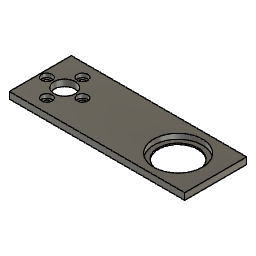
sample stage arm (Autodesk Fusion 360 design; units mm, degrees)
Autodesk Fusion 360 part; units mm, degrees
box "BoxPrimitive1" add length 47 width 105 height 5 placed x (0, -1, 0) y (1, 0, 0) z (0, 0, 1) at (0, 0, 0) makes body 1
cylinder "CylinderPrimitive2" add diameter 8 height 3 placed x (1, 0, 0) y (0, 1, 0) z (0, 0, 1) at (0, 0, 0) separate body makes body 2
move_body "Move1" bodies 2 to x (1, 0, 0) y (0, 1, 0) z (0, 0, 1) at (8, -23.5, 5)
copy_body "CopyPasteBodies1" bodies 2 makes body 3
move_body "Move2" bodies 3 to x (1, 0, 0) y (0, 1, 0) z (0, 0, 1) at (27, 0, 0)
copy_body "CopyPasteBodies2" bodies 3 makes body 4
move_body "Move3" bodies 4 to x (1, 0, 0) y (0, 1, 0) z (0, 0, 1) at (-13.5, 13.5, 0)
copy_body "CopyPasteBodies3" bodies 4 makes body 5
move_body "Move4" bodies 5 to x (1, 0, 0) y (0, 1, 0) z (0, 0, 1) at (0, -27, 0)
move_body "Move5" bodies 4 to x (1, 0, 0) y (0, 1, 0) z (0, 0, 1) at (0, 0, -3)
move_body "Move6" bodies 3 to x (1, 0, 0) y (0, 1, 0) z (0, 0, 1) at (0, 0, -3)
move_body "Move7" bodies 5 to x (1, 0, 0) y (0, 1, 0) z (0, 0, 1) at (0, 0, -3)
move_body "Move8" bodies 2 to x (1, 0, 0) y (0, 1, 0) z (0, 0, 1) at (0, 0, -3)
combine "Combine1" operation cut target body 1 tool bodies 4 3 5 2
cylinder "CylinderPrimitive3" add diameter 4.5 height 2 placed x (1, 0, 0) y (0, 1, 0) z (0, 0, 1) at (21.5, -10, 2) separate body makes body 6
cylinder "CylinderPrimitive4" add diameter 4.5 height 2 placed x (1, 0, 0) y (0, 1, 0) z (0, 0, 1) at (35, -23.5, 2) separate body makes body 7
cylinder "CylinderPrimitive5" add diameter 4.5 height 2 placed x (1, 0, 0) y (0, 1, 0) z (0, 0, 1) at (8, -23.5, 2) separate body makes body 8
cylinder "CylinderPrimitive6" add diameter 4.5 height 2 placed x (1, 0, 0) y (0, 1, 0) z (0, 0, 1) at (21.5, -37, 2) separate body makes body 9
move_body "Move9" bodies 6 to x (1, 0, 0) y (0, 1, 0) z (0, 0, 1) at (0, 0, -2)
move_body "Move10" bodies 8 to x (1, 0, 0) y (0, 1, 0) z (0, 0, 1) at (0, 0, -2)
move_body "Move11" bodies 7 to x (1, 0, 0) y (0, 1, 0) z (0, 0, 1) at (0, 0, -2)
move_body "Move12" bodies 9 to x (1, 0, 0) y (0, 1, 0) z (0, 0, 1) at (0, 0, -2)
combine "Combine2" operation cut target body 1 tool bodies 6 7 8 9
cylinder "CylinderPrimitive7" add diameter 16 height 5 placed x (1, 0, 0) y (0, 1, 0) z (0, 0, 1) at (0, 0, 0) separate body makes body 10
move_body "Move14" bodies 10 to x (1, 0, 0) y (0, 1, 0) z (0, 0, 1) at (21.5, -23.5, 0)
combine "Combine3" operation cut target body 1 tool bodies 10
box "BoxPrimitive3" cut length 47 width 3 height 5 placed x (0, -1, 0) y (1, 0, 0) z (0, 0, 1) at (0, 0, 0) bodies 1
cylinder "CylinderPrimitive8" add diameter 37 height 4 placed x (1, 0, 0) y (0, 1, 0) z (0, 0, 1) at (0, 0, 5) separate body makes body 11
move_body "Move16" bodies 11 to x (1, 0, 0) y (0, 1, 0) z (0, 0, 1) at (76, -25, -3)
move_body "Move19" bodies 11 to x (1, 0, 0) y (0, 1, 0) z (0, 0, 1) at (0, 25, 0)
box "BoxPrimitive4" add length 47 width 20 height 5 placed x (0, -1, 0) y (1, 0, 0) z (0, 0, 1) at (0, 0, 0) separate body makes body 12
move_body "Move20" bodies 12 to x (1, 0, 0) y (0, 1, 0) z (0, 0, 1) at (105, 0, 0)
combine "Combine7" operation add target body 12 tool bodies 1
move_body "Move21" bodies 11 to x (1, 0, 0) y (0, 1, 0) z (0, 0, 1) at (20, -23.5, 0)
cylinder "CylinderPrimitive10" add diameter 30 height 2 placed x (1, 0, 0) y (0, 1, 0) z (0, 0, 1) at (0, 0, 5) separate body makes body 13
move_body "Move22" bodies 11 to x (1, 0, 0) y (0, 1, 0) z (0, 0, 1) at (11.5, 0, 0)
box "BoxPrimitive5" add length 47 width 11.357 height 5 placed x (0, -1, 0) y (1, 0, 0) z (0, 0, 1) at (0, 0, 0) separate body makes body 14
move_body "Move23" bodies 14 to x (1, 0, 0) y (0, 1, 0) z (0, 0, 1) at (125, 0, 0)
combine "Combine9" operation add target body 14 tool bodies 12
box "BoxPrimitive6" add length 47 width 0.357 height 5 placed x (0, -1, 0) y (1, 0, 0) z (0, 0, 1) at (0, 0, 0) separate body makes body 15
move_body "Move24" bodies 15 to x (1, 0, 0) y (0, 1, 0) z (0, 0, 1) at (136, 0, 0)
combine "Combine10" operation cut target body 14 tool bodies 15
move_body "Move25" bodies 13 to x (1, 0, 0) y (0, 1, 0) z (0, 0, 1) at (107.5, -23.5, -5)
move_body "Move26" bodies 11 to x (1, 0, 0) y (0, 1, 0) z (0, 0, 1) at (0, 0, -1)
combine "Combine13" operation cut target body 14 tool bodies 11
combine "Combine14" operation cut target body 14 tool bodies 13
